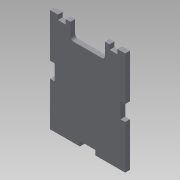
# Autodesk Inventor part: Top
Saved by Autodesk Inventor 2013 (Build 170138000, 138)
## iProperties
Created: 2013-12-12
Part Number: Top
Material: Generic
Document SubType Name: Modeling
Designer: Eric
Density: 1 g/cm^3
Author: Eric
Autodesk Inventor part; units mm, degrees
ref_plane "YZ Plane" through (0, 0, 0) normal (1, 0, 0) x (0, 1, 0)
ref_plane "XZ Plane" through (0, 0, 0) normal (0, 1, 0) x (-1, 0, 0)
ref_plane "XY Plane" through (0, 0, 0) normal (0, 0, 1) x (1, 0, 0)
sketch "Sketch1" plane through (0, 0, 0) normal (0, 1, 0) x (-1, 0, 0)
  line L0 (19, 0) -> (19, 3)
  line L1 (19, 3) -> (29, 3)
  line L2 (29, 3) -> (29, 0)
  line L3 (0, 0) -> (19, 0)
  line L4 (29, 0) -> (48, 0)
  line L5 (0, 66) -> (0, 38)
  line L6 (0, 28) -> (0, 0)
  line L7 (48, 0) -> (48, 28)
  line L8 (48, 38) -> (48, 66)
  line L9 (0, 38) -> (3, 38)
  line L10 (3, 38) -> (3, 28)
  line L11 (3, 28) -> (0, 28)
  line L12 (48, 38) -> (45, 38)
  line L13 (45, 38) -> (45, 28)
  line L14 (45, 28) -> (48, 28)
  line L15 (5, 66) -> (5, 63)
  line L16 (5, 63) -> (10, 63)
  line L17 (10, 63) -> (10, 66)
  line L18 (38, 66) -> (38, 63)
  line L19 (38, 63) -> (43, 63)
  line L20 (43, 63) -> (43, 66)
  line L21 (0, 66) -> (5, 66)
  line L22 (43, 66) -> (48, 66)
  line L23 (13, 66) -> (13, 58)
  line L24 (15, 56) -> (33, 56)
  line L25 (35, 58) -> (35, 66)
  line L26 (10, 66) -> (13, 66)
  line L27 (35, 66) -> (38, 66)
  arc A0 (13, 58) -> (15, 56) centre (15, 58) ccw
  arc A1 (33, 56) -> (35, 58) centre (33, 58) ccw
  point P0 (13, 56)
  point P1 (35, 56)
  dimension "d8" = 3
  dimension "d9" = 3
  dimension "d22" = 19
  dimension "d23" = 3
  dimension "d24" = 10
  dimension "d25" = 10
  dimension "d26" = 3
  dimension "d27" = 28
  dimension "d28" = 28
  dimension "d29" = 3
  dimension "d30" = 3
  dimension "d31" = 19
  dimension "d35" = 3
  dimension "d36" = 3
  dimension "d37" = 3
  dimension "d38" = 3
  dimension "d39" = 5
  dimension "d41" = 5
  dimension "d42" = 5
  dimension "d43" = 28
  dimension "d44" = 28
  dimension "d48" = 10
  dimension "d49" = 2
  dimension "d50" = 48
  dimension "d51" = 5
  dimension "d52" = 13
  dimension "d53" = 13
  constraints: 56 end point, 28 perpendicular, 12 parallel, 4 point on circle, 4 point on line, 4 tangent, 2 centre point, 2 horizontal, 1 equal radius
  measures "d8" distance of L0.start L0.end
  measures "d9" distance of L1.end L2.end
  measures "d22" distance of L3.start L0.start
  measures "d23" distance of L5.end L9.end
  measures "d24" distance of L9.end L10.end
  measures "d25" distance of L12.end L13.end
  measures "d26" distance of L8.start L12.end
  measures "d27" distance of L6.start L3.start
  measures "d28" distance of L4.end L7.end
  measures "d29" distance of L10.end L6.start
  measures "d30" distance of L13.end L7.end
  measures "d31" distance of L2.end L4.end
  measures "d35" distance of L15.start L15.end
  measures "d36" distance of L16.end L17.end
  measures "d37" distance of L18.start L18.end
  measures "d38" distance of L19.end L20.end
  measures "d39" distance between parallel lines of L5 L15
  measures "d41" distance of L18.end L19.end
  measures "d42" distance of L15.end L16.end
  measures "d43" distance of L5.start L5.end
  measures "d44" distance of L8.start L8.end
  measures "d48" distance of L23.start point (13, 56)
  measures "d49" radius of A0
  measures "d50" distance between parallel lines of L8 L5
  measures "d51" distance of L20.end L8.end
  measures "d52" distance between parallel lines of L5 L23
  measures "d53" distance between parallel lines of L8 L25
extrude "Extrusion1" add sketch "Sketch1" along normal blind 3
body "Solid1"
